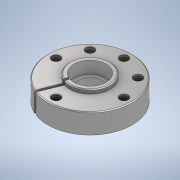
# Autodesk Inventor part: OutputHorn
Saved by Autodesk Inventor 2020 (Build 240168000, 168)
## iProperties
Created: 2021-08-24
Part Number: OutputHorn
Material: 一般
Document SubType Name: Modeling
Designer: naoki
Density: 1 g/cm^3
Appearance: ステンレス - ブラシ仕上げ
Description: 既製品
Author: naoki
Autodesk Inventor part; units mm, degrees
ref_plane "YZ Plane" through (0, 0, 0) normal (1, 0, 0) x (0, 1, 0)
ref_plane "XZ Plane" through (0, 0, 0) normal (0, 1, 0) x (-1, 0, 0)
ref_plane "XY Plane" through (0, 0, 0) normal (0, 0, 1) x (1, 0, 0)
sketch "スケッチ1" plane through (0, 0, 0) normal (0, 1, 0) x (-1, 0, 0)
  line L0 (0, 0) -> (6.3, 0)
  line L1 (6.3, -5) -> (6.3, -10.5)
  line L2 (6.3, -10.5) -> (1.3, -10.5)
  line L3 (1.3, -10.5) -> (1.3, -4)
  line L4 (6.3, -5) -> (7.3, -5)
  line L5 (7.3, -5) -> (7.3, -4)
  line L6 (7.3, -4) -> (4.25, -4)
  line L7 (4.25, -4) -> (4.25, -3)
  line L8 (4.25, -3) -> (0, -3)
  line L9 (1.3, -4) -> (0, -4)
  line L10 (0, -4) -> (0, -3)
  line L11 (0, -3) -> (0, -3)
  point P0 (0, -3)
  dimension "d0" = 5
  dimension "d1" = 10.5
  dimension "d16" = 3.05
  dimension "d18" = 3
  dimension "d22" = 1.3
  dimension "d31" = 5
  dimension "d32" = 4
  dimension "d33" = 1
  dimension "d34" = 4
  constraints: 24 end point, 6 perpendicular, 2 horizontal, 2 parallel, 2 point on line
  measures "d0" distance of L1.end L2.end
  measures "d1" distance of L0.end L1.end
  measures "d16" distance of L5.end L6.end
  measures "d18" distance between parallel lines of L0 L8
  measures "d22" distance of L3.end L9.end
  measures "d31" distance between parallel lines of L0 L4
  measures "d32" distance between parallel lines of L0 L9
  measures "d33" horizontal distance of L4.end L1.end
  measures "d34" distance between parallel lines of L0 L6
revolve "回転1" add sketch "スケッチ1" angle 360 about axis through (0, 0, 0) along (-1, 0, 0)
sketch "スケッチ2" plane through (-6.3, 0, 0) normal (-1, 0, 0) x (0, 0, 1)
  line L0 (14.2354, 0) -> (-14.2704, 0) construction
  line L1 (-0.0175, -14.7426) -> (-0.0175, 15.0224) construction
  point P0 (0, 0)
  point P1 (0, -8.5)
  dimension "d5" = 8.5
  constraints: 4 end point, 1 horizontal, 1 vertical
  measures "d5" distance of point (0, -8.5) point (0, 0)
hole "穴1" at (-6.3, -8.5, 0) direction (1, 0, 0) diameter 2.1129 end through all thread size "M2.6x0.45" class "6H" standard "ANSI Metric M Profile"
pattern_circular "円形状パターン1" count 8 over 360 about axis through (-6.8, 0, 0) along (1, 0, 0) of "穴1" skipped copies 6 8
chamfer "面取り1" distance 0.2 angle 45 3 edges at (-7.3, 0, 5) (-6.3, 0, 10.5) (0, 0, 4)
sketch "スケッチ3" plane through (-7.3, 0, 0) normal (-1, 0, 0) x (0, 0, 1)
  circle A0 centre (0, 0) radius 10.5 projected
  line L0 (9.8478, -3.6552) -> (0.1124, 0.2782)
  line L1 (9.623, -4.2115) -> (-0.1124, -0.2782)
  line L2 (9.623, -4.2115) -> (9.8478, -3.6552)
  line L3 (-0.1124, -0.2782) -> (0.1124, 0.2782)
  line L4 (14.8528, 0) -> (-19.4242, 0) construction
  point P0 (0.1068, 0.2803)
  point P1 (9.6191, -4.2099)
  point P2 (9.8438, -3.6536)
  dimension "d25" = 10.5
  dimension "d26" = 0.6
  dimension "d27" = 0.3
  dimension "d30" = 22
  constraints: 10 end point, 3 point on line, 2 perpendicular, 1 horizontal
  measures "d25" distance of L1.start L1.end
  measures "d26" distance between parallel lines of L0 L1
  measures "d27" distance from line of point (0, 0) L1
  measures "d30" angle of L0 L4
extrude "押し出し1" cut sketch "スケッチ3" against normal up to surface (7.3 mm away) contours L1 L3 L0 A0 picked at (3.2451, -1.3113)
